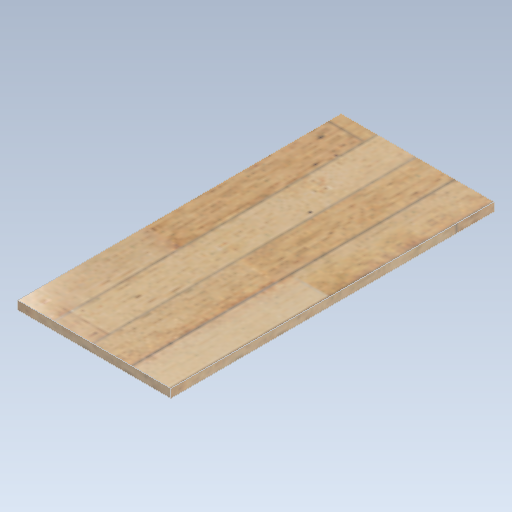
# Autodesk Inventor part: Creat Buttom-01
Saved by Autodesk Inventor 2021 (Build 250183000, 183)
## iProperties
Created: 2020-08-15
Part Number: Creat Buttom-01
Material: Wood (Maple)
Document SubType Name: Modeling
Designer: Oghenemarho
Density: 0.67 g/cm^3
Appearance: Natural Maple - Glossy Dark Tint
Mass: 595.635 g
Surface Area: 2898.4 cm^2
Volume: 889.008 cm^3
Author: Oghenemarho
Autodesk Inventor part; units mm, degrees
ref_plane "YZ Plane" through (0, 0, 0) normal (1, 0, 0) x (0, 1, 0)
ref_plane "XZ Plane" through (0, 0, 0) normal (0, 1, 0) x (-1, 0, 0)
ref_plane "XY Plane" through (0, 0, 0) normal (0, 0, 1) x (1, 0, 0)
sketch "Sketch1" plane through (0, 0, 0) normal (0, 1, 0) x (-1, 0, 0)
  line L0 (-112.3, 237.3) -> (112.3, 237.3)
  line L1 (112.3, 237.3) -> (112.3, -237.3)
  line L2 (112.3, -237.3) -> (-112.3, -237.3)
  line L3 (-112.3, -237.3) -> (-112.3, 237.3)
  line L4 (-112.3, 237.3) -> (112.3, -237.3) construction
  line L5 (112.3, 237.3) -> (-112.3, -237.3) construction
  point P0 (0, 0)
  dimension "Width" = 224.6
  dimension "lenght" = 474.6
  constraints: 12 end point, 2 midpoint, 2 parallel, 1 horizontal, 1 perpendicular
  measures "Width" distance of L1.end L2.end
  measures "lenght" distance of L2.end L0.start
extrude "Extrusion1" add sketch "Sketch1" along normal blind 12.7
body "Solid1"
